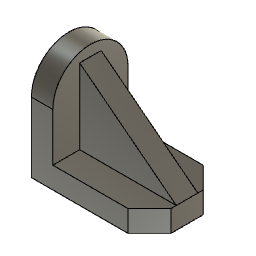
A1 v1 (Autodesk Fusion 360 design; units mm, degrees)
Autodesk Fusion 360 part; units mm, degrees
sketch "bottom" plane through (0, 0, 0) normal (0, 0, 1) x (1, 0, 0)
  line L0 (33, 21) -> (-33, 21)
  line L1 (-33, 21) -> (-33, -21)
  line L2 (-33, -21) -> (33, -21)
  line L3 (33, -21) -> (33, 21)
  line L4 (33, 21) -> (-33, -21) construction
  line L5 (-33, 21) -> (33, -21) construction
  dimension "d32" = 66
  dimension "d33" = 42
  constraint horizontal L0
  constraint perpendicular L0 L1
  constraint parallel L0 L2
  constraint parallel L1 L3
  constraint coincident L4 origin
  constraint coincident L5 origin
  measures "d32" distance of L0.start L0.end
  measures "d33" distance of L0.end L1.end
extrude "Extrude7" add sketch "bottom" along normal blind 12
chamfer "Chamfer1" distance 12 angle 45 1 edges at (33, -21, 6)
chamfer "Chamfer2" distance 12 angle 45 1 edges at (33, 21, 6)
sketch "wall" plane through (0, 0, 12) normal (0, 0, 1) x (-1, 0, 0)
  line L0 (-33, -9) -> (-21, -21)
  line L1 (-21, -21) -> (33, -21)
  line L2 (33, -21) -> (33, 21)
  line L3 (33, 21) -> (-21, 21)
  line L4 (-21, 21) -> (-33, 9)
  line L5 (-33, 9) -> (-33, -9)
  line L6 (33, -21) -> (21, -21)
  line L7 (21, -21) -> (21, 21)
  line L8 (21, 21) -> (33, 21)
  line L9 (33, 21) -> (33, -21)
  dimension "d38" = 12
  constraint horizontal L6
  constraint vertical L7
  constraint horizontal L8
  constraint vertical L9
  constraint coincident L3 L7.end
  constraint coincident L1.end L2.start
  measures "d38" distance of L1.end L6.end
extrude "Extrude8" add sketch "wall" along normal blind 60 contours L1 L2 L3 L6 L7 L8 L9
extrude "Extrude9" cut 1 faces at (-29, 7, 72) along direction (0, 0, -1) blind 12
fillet "Fillet1" radius 21 2 edges at (-27, -21, 60) (-27, 21, 60)
sketch "Sketch10" plane through (0, 0, 0) normal (0, 1, 0) x (1, 0, 0)
  line L0 (-21, -12) -> (-21, -54)
  line L1 (-21, -54) -> (33, -12)
  line L2 (33, -12) -> (-21, -12)
  dimension "d45" = 42
  dimension "d46" = 54
  constraint vertical L0
  constraint perpendicular L0 L2
  measures "d45" distance of L0.start L0.end
  measures "d46" distance of L0.start L1.end
extrude "Extrude10" add sketch "Sketch10" along normal mid plane 12
